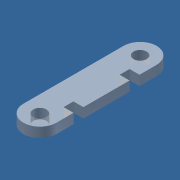
# Autodesk Inventor part: orejapress
Saved by Autodesk Inventor 2014 (Build 180170000, 170)
## iProperties
Created: 2013-09-11
Part Number: orejapress
Material: Glass
Document SubType Name: Modeling
Designer: Lefo
Density: 2.18 g/cm^3
Appearance: Clear
Author: Lefo
Autodesk Inventor part; units mm, degrees
ref_plane "YZ Plane" through (0, 0, 0) normal (1, 0, 0) x (0, 1, 0)
ref_plane "XZ Plane" through (0, 0, 0) normal (0, 1, 0) x (-1, 0, 0)
ref_plane "XY Plane" through (0, 0, 0) normal (0, 0, 1) x (1, 0, 0)
sketch "Sketch1" plane through (0, 0, 0) normal (0, 1, 0) x (-1, 0, 0)
  line L0 (11.2248, 8.7019) -> (21.2248, 8.7019)
  line L1 (21.2248, 8.7019) -> (21.2248, 13.9019)
  line L2 (11.2248, 13.9019) -> (11.2248, 8.7019)
  arc A0 (16.2248, 18.9019) -> (11.2248, 13.9019) centre (16.2248, 13.9019) ccw
  arc A1 (21.2248, 13.9019) -> (16.2248, 18.9019) centre (16.2248, 13.9019) ccw
  circle A2 centre (16.2248, 13.9019) radius 2
  line L3 (13.7248, 8.7019) -> (18.7248, 8.7019)
  point P0 (21.2248, 18.9019)
  point P1 (11.2248, 18.9019)
  dimension "d0" = 10
  dimension "d1" = 10.2
  dimension "d7" = 5
  dimension "d8" = 4
  constraints: 8 end point, 4 point on circle, 3 centre point, 3 horizontal, 3 point on line, 2 coincident, 2 tangent, 1 concentric, 1 parallel, 1 perpendicular, 7 other
  measures "d0" distance of point (11.225, 18.902) point (21.225, 18.902)
  measures "d1" distance of point (21.225, 18.902) L0.end
  measures "d7" radius of A0
  measures "d8" diameter of A2
extrude "Extrusion1" add sketch "Sketch1" along normal blind 3
sketch "Sketch2" plane through (-11.2248, 0, 8.7019) normal (0, 0, -1) x (-1, 0, 0)
  line L0 (10, 0) -> (0, 0) projected
  line L1 (10, 0) -> (10, 3) projected
  line L2 (0, 3) -> (10, 3) projected
  line L3 (0, 0) -> (0, 3) projected
  point P0 (-11.2248, 0)
extrude "Extrusion2" add sketch "Sketch2" along normal blind 30.2
fillet "Fillet1" radius 5 2 edges at (-21.2248, 1.5, -21.4981) (-11.2248, 1.5, -21.4981)
hole "Hole1" at (-16.2248, 3, -16.4981) direction (0, -1, 0) diameter 4 depth 3
sketch "Sketch3" plane through (0, 0, 0) normal (0, -1, 0) x (1, 0, 0)
  line L0 (-11.2248, -16.4981) -> (-11.2248, 13.9019) projected
  line L1 (-21.2248, 13.9019) -> (-21.2248, -16.4981) projected
  line L2 (-14.2248, 8.7019) -> (-11.2248, 8.7019)
  line L3 (-11.2248, 8.7019) -> (-11.2248, 5.7019)
  line L4 (-11.2248, 5.7019) -> (-14.2248, 5.7019)
  line L5 (-14.2248, 5.7019) -> (-14.2248, 8.7019)
  line L6 (-11.2248, -1.2981) -> (-21.2248, -1.2981) construction
  line L7 (-14.2248, -11.2981) -> (-11.2248, -11.2981)
  line L8 (-11.2248, -11.2981) -> (-11.2248, -8.2981)
  line L9 (-11.2248, -8.2981) -> (-14.2248, -8.2981)
  line L10 (-14.2248, -8.2981) -> (-14.2248, -11.2981)
  point P0 (0, 0)
  dimension "d28" = 3
  dimension "d29" = 3
  dimension "d33" = 7
  constraints: 18 end point, 4 symmetric about line, 2 midpoint, 2 parallel, 1 collinear, 1 horizontal, 1 perpendicular
  measures "d28" distance of L3.end L4.end
  measures "d29" distance of L2.end L3.end
  measures "d33" distance between parallel lines of L6 L4
extrude "Extrusion3" cut sketch "Sketch3" against normal up to next
body "Solid1"
